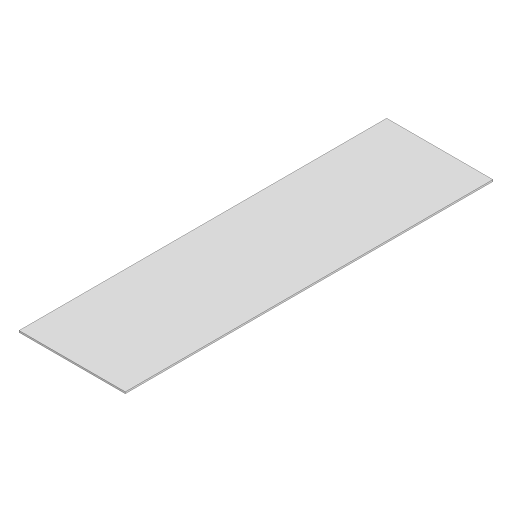
# Autodesk Inventor part: CANALETA_PLANA
Saved by Autodesk Inventor 2024 (Build 280153000, 153)
## iProperties
Created: 2024-08-15
Part Number: CANALETA_PLANA
Material: Generic
Document SubType Name: Modeling
Designer: Jhuliams
Density: 1 g/cm^3
Appearance: Default
Author: Jhuliams
Autodesk Inventor part; units mm, degrees
ref_plane "YZ Plane" through (0, 0, 0) normal (1, 0, 0) x (0, 1, 0)
ref_plane "XZ Plane" through (0, 0, 0) normal (0, 1, 0) x (-1, 0, 0)
ref_plane "XY Plane" through (0, 0, 0) normal (0, 0, 1) x (1, 0, 0)
sketch "Sketch1" plane through (0, 0, 0) normal (0, 1, 0) x (-1, 0, 0)
  line L0 (65, 225) -> (-65, 225)
  line L1 (-65, 225) -> (-65, -225)
  line L2 (-65, -225) -> (65, -225)
  line L3 (65, -225) -> (65, 225)
  line L4 (65, 225) -> (-65, -225) construction
  line L5 (-65, 225) -> (65, -225) construction
  point P0 (0, 0)
  dimension "d0" = 130
  dimension "d1" = 450
  constraints: 12 end point, 2 midpoint, 2 parallel, 1 horizontal, 1 perpendicular
  measures "d0" distance of L2.end L1.end
  measures "d1" distance of L1.end L0.end
extrude "Extrusion1" add sketch "Sketch1" along normal blind 2
body "Solid1"
